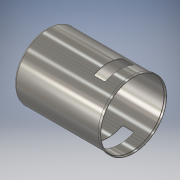
# Autodesk Inventor part: Motor-Casing
Saved by Autodesk Inventor 2016 (Build 200138000, 138)
## iProperties
Created: 2015-05-19
Part Number: Motor-Casing
Material: Generic
Document SubType Name: Modeling
Designer: jonathan
Density: 1 g/cm^3
Appearance: Steel - Polished
Mass: 1.51152 g
Surface Area: 119.61 cm^2
Volume: 1.51152 cm^3
Author: jonathan
Autodesk Inventor part; units mm, degrees
ref_plane "YZ Plane" through (0, 0, 0) normal (1, 0, 0) x (0, 1, 0)
ref_plane "XZ Plane" through (0, 0, 0) normal (0, 1, 0) x (-1, 0, 0)
ref_plane "XY Plane" through (0, 0, 0) normal (0, 0, 1) x (1, 0, 0)
sketch "Sketch1" plane through (0, 0, 0) normal (1, 0, 0) x (0, 1, 0)
  circle A0 centre (0, 0) radius 17.78
  dimension "d0" = 35.56
  constraints: 1 centre point, 1 coincident
  measures "d0" diameter of A0
extrude "Extrusion1" add sketch "Sketch1" along normal blind 47.625
fillet "Fillet1" radius 1.27 1 edges at (0, -17.78, 0)
sketch "Sketch2" plane through (0, 0, 0) normal (0, 1, 0) x (-1, 0, 0)
  line L0 (-34.29, -7.9375) -> (-39.37, -7.9375)
  line L1 (-40.005, -7.3025) -> (-40.005, 7.3025)
  line L2 (-39.37, 7.9375) -> (-34.29, 7.9375)
  line L3 (-33.655, 7.3025) -> (-33.655, -7.3025)
  line L4 (-47.625, 17.78) -> (-47.625, -17.78) projected
  arc A0 (-40.005, -7.3025) -> (-39.37, -7.9375) centre (-39.37, -7.3025) ccw
  arc A1 (-34.29, -7.9375) -> (-33.655, -7.3025) centre (-34.29, -7.3025) ccw
  arc A2 (-33.655, 7.3025) -> (-34.29, 7.9375) centre (-34.29, 7.3025) ccw
  arc A3 (-39.37, 7.9375) -> (-40.005, 7.3025) centre (-39.37, 7.3025) ccw
  point P0 (0, 0)
  point P1 (-33.655, -7.9375)
  point P2 (-40.005, 7.9375)
  point P3 (-40.005, -7.9375)
  point P4 (-33.655, 7.9375)
  dimension "d4" = 15.875
  dimension "d5" = 6.35
  dimension "d6" = 7.62
  dimension "d7" = 9.8425
  dimension "d14" = 0.635
  constraints: 8 end point, 8 point on circle, 8 point on line, 8 tangent, 4 centre point, 3 equal radius, 2 parallel, 1 horizontal, 1 perpendicular
  measures "d4" distance of point (-40.005, -7.937) point (-40.005, 7.938)
  measures "d5" distance of point (-40.005, 7.938) point (-33.655, 7.938)
  measures "d6" distance from line of point (-40.005, -7.937) L4
  measures "d7" distance from line of L0 L4.end
  measures "d14" radius of A0
sketch "Sketch3" plane through (47.625, 0, 0) normal (1, 0, 0) x (0, 0, -1)
  circle A0 centre (0, 0) radius 18.0975
  dimension "d11" = 36.195
  constraints: 1 centre point, 1 coincident
  measures "d11" diameter of A0
extrude "Extrusion3" add sketch "Sketch3" against normal blind 1.27
shell "Shell2" thickness 0.254 removed faces 1 at (47.625, -0.1965, 3.481)
extrude "Extrusion2" cut sketch "Sketch2" along normal up to next
sketch "Sketch4" plane through (0, 0, 0) normal (-1, 0, 0) x (0, 0, 1)
  circle A0 centre (0, 0) radius 4.7625
  dimension "d16" = 9.525
  constraints: 1 centre point, 1 coincident
  measures "d16" diameter of A0
extrude "Extrusion4" cut sketch "Sketch4" against normal up to next
extrude "Extrusion5" cut sketch "Sketch2" against normal up to next
body "Solid1"
